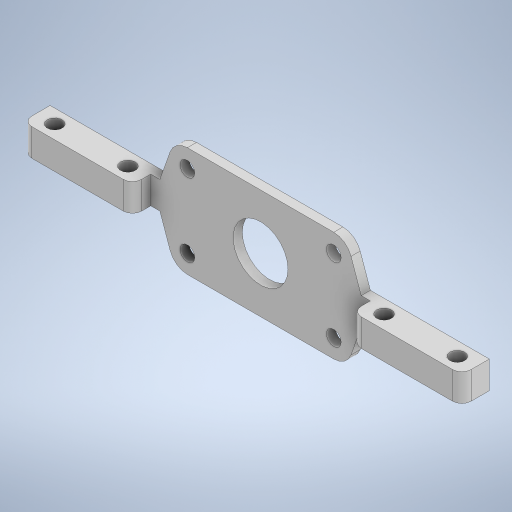
# Autodesk Inventor part: Face Plate
Saved by Autodesk Inventor 2023 (Build 270158000, 158)
## iProperties
Created: 2023-02-27
Part Number: Face Plate
Material: Generic
Document SubType Name: Modeling
Designer: Gabriel - T3 CAD
Density: 1 g/cm^3
Appearance: Default
Author: Gabriel - T3 CAD
Autodesk Inventor part; units mm, degrees
ref_plane "YZ Plane" through (0, 0, 0) normal (1, 0, 0) x (0, 1, 0)
ref_plane "XZ Plane" through (0, 0, 0) normal (0, 1, 0) x (-1, 0, 0)
ref_plane "XY Plane" through (0, 0, 0) normal (0, 0, 1) x (1, 0, 0)
sketch "Sketch1" plane through (0, 0, 0) normal (0, 1, 0) x (-1, 0, 0)
  line L0 (0, 0) -> (152.4, 0)
  line L1 (152.4, 0) -> (152.4, 6.35)
  line L2 (34.925, 9.525) -> (3.175, 9.525)
  line L3 (0, 6.35) -> (0, 0)
  circle A0 centre (6.35, 4.7625) radius 2.5797
  circle A1 centre (31.75, 4.7625) radius 2.5797
  circle A2 centre (120.65, 4.7625) radius 2.5797
  circle A3 centre (146.05, 4.7625) radius 2.5797
  line L4 (38.1, 9.525) -> (114.3, 9.525)
  line L5 (114.3, 6.35) -> (114.3, 4.7625)
  line L6 (38.1, 4.7625) -> (38.1, 6.35)
  arc A4 (38.1, 6.35) -> (34.925, 9.525) centre (34.925, 6.35) ccw
  arc A5 (3.175, 9.525) -> (0, 6.35) centre (3.175, 6.35) ccw
  line L7 (117.475, 9.525) -> (149.225, 9.525)
  arc A6 (117.475, 9.525) -> (114.3, 6.35) centre (117.475, 6.35) ccw
  arc A7 (152.4, 6.35) -> (149.225, 9.525) centre (149.225, 6.35) ccw
  line L8 (114.3, 6.35) -> (114.3, 0)
  line L9 (38.1, 6.35) -> (38.1, 0)
  line L10 (114.3, 4.7625) -> (114.3, 9.525)
  line L11 (117.475, 9.525) -> (114.3, 9.525)
  line L12 (38.1, 6.35) -> (38.1, 9.525)
  line L13 (38.1, 9.525) -> (34.925, 9.525)
  line L14 (38.1, 3.175) -> (114.3, 3.175)
  point P0 (152.4, 9.525)
  point P1 (0, 9.525)
  dimension "d0" = 152.4
  dimension "d1" = 9.525
  dimension "d2" = 4.7625
  dimension "d3" = 4.7625
  dimension "d4" = 4.7625
  dimension "d5" = 4.7625
  dimension "d6" = 25.4
  dimension "d7" = 25.4
  dimension "d8" = 5.1594
  dimension "d9" = 6.35
  dimension "d10" = 6.35
  dimension "d11" = 4.7625
  dimension "d12" = 6.35
  dimension "d13" = 6.35
  dimension "d14" = 3.175
  dimension "d15" = 3.175
  dimension "d37" = 3.175
  constraints: 30 end point, 11 point on line, 10 tangent, 8 centre point, 8 point on circle, 7 perpendicular, 5 equal radius, 3 horizontal, 3 parallel, 2 midpoint
  measures "d0" distance of point (152.4, 9.525) point (0, 9.525)
  measures "d1" distance of L0.end point (152.4, 9.525)
  measures "d2" distance from line of L0 A0.centre
  measures "d3" distance from line of L0 A1.centre
  measures "d4" distance from line of L0 A2.centre
  measures "d5" distance from line of L0 A3.centre
  measures "d6" distance of A0.centre A1.centre
  measures "d7" distance of A2.centre A3.centre
  measures "d8" diameter of A3
  measures "d9" distance from line of L3 A0.centre
  measures "d10" distance from line of L1 A3.centre
  measures "d11" distance of L6.start L4.start
  measures "d12" distance from line of A1.centre L6
  measures "d13" distance from line of A2.centre L5
  measures "d14" radius of A4
  measures "d15" radius of A6
  measures "d37" distance between parallel lines of L14 L0
extrude "Extrusion1" add sketch "Sketch1" along normal mid plane 9.525 contours L3 A5 L2 A4 L6 L9 L0 | L9 L14 L8 L0 | L8 L5 A6 L7 A7 L1 L0
extrude "Extrusion2" add sketch "Sketch1" along normal mid plane 50.8 contours L9 L14 L8 L0
sketch "Sketch3" plane through (-152.4, -4.7625, 0) normal (0, 0, -1) x (-1, 0, 0)
  line L0 (-38.1, -20.6375) -> (-38.1, 0)
  line L1 (-114.3, 30.1625) -> (-38.1, 30.1625)
  line L2 (-38.1, 30.1625) -> (-38.1, -20.6375)
  line L3 (-38.1, -20.6375) -> (-114.3, -20.6375)
  line L4 (-114.3, -20.6375) -> (-114.3, 30.1625)
  circle A0 centre (-76.2, 4.7625) radius 9.525
  line L5 (-101.6, -20.6375) -> (-101.6, 30.1625)
  line L6 (-101.6, 30.1625) -> (-50.8, 30.1625)
  line L7 (-50.8, 30.1625) -> (-50.8, -20.6375)
  line L8 (-50.8, -20.6375) -> (-101.6, -20.6375)
  line L9 (-101.6, 17.4625) -> (-50.8, 17.4625)
  line L10 (-50.8, 17.4625) -> (-50.8, -7.9375)
  line L11 (-50.8, -7.9375) -> (-101.6, -7.9375)
  line L12 (-101.6, -7.9375) -> (-101.6, 17.4625)
  circle A1 centre (-101.6, 17.4625) radius 2.5797
  circle A2 centre (-101.6, -7.9375) radius 2.5797
  circle A3 centre (-50.8, -7.9375) radius 2.5797
  circle A4 centre (-50.8, 17.4625) radius 2.5797
  circle A5 centre (-101.6, 17.4625) radius 6.35
  circle A6 centre (-101.6, -7.9375) radius 6.35
  circle A7 centre (-50.8, -7.9375) radius 6.35
  circle A8 centre (-50.8, 17.4625) radius 6.35
  line L13 (-107.95, 23.8125) -> (-44.45, 23.8125)
  line L14 (-44.45, 23.8125) -> (-44.45, -14.2875)
  line L15 (-44.45, -14.2875) -> (-107.95, -14.2875)
  line L16 (-107.95, -14.2875) -> (-107.95, 23.8125)
  line L17 (-114.3, 9.525) -> (-117.475, 9.525)
  line L18 (-114.3, 0) -> (-114.3, 9.525)
  line L19 (-38.1, 0) -> (-38.1, 9.525)
  line L20 (-114.3, 9.525) -> (-107.95, 9.525)
  line L21 (-111.125, 9.525) -> (-101.3931, 37.1795)
  line L22 (-114.3, 0) -> (-114.3, 9.525)
  line L23 (-114.3, 0) -> (-107.95, 0)
  line L24 (-111.125, 0) -> (-100.7566, -29.4634)
  line L25 (-38.1, 0) -> (-44.45, 0)
  line L26 (-38.1, 9.525) -> (-38.1, 30.1625)
  line L27 (-38.1, 9.525) -> (-44.45, 9.525)
  line L28 (-41.275, 9.525) -> (-52.247, 40.7036)
  line L29 (-41.275, 0) -> (-51.6214, -29.4007)
  line L30 (0, 0) -> (-38.1, 0) projected
  line L31 (-114.3, 9.525) -> (-114.3, 30.1625) projected
  point P0 (-152.4, 4.7625)
  point P1 (-41.275, 0)
  point P2 (-107.5899, 19.5704)
  point P3 (-101.6, 23.8125)
  point P4 (-50.8, 23.8125)
  point P5 (-44.8101, 19.5704)
  point P6 (-38.1, 0)
  point P7 (-44.8101, -10.0454)
  point P8 (-50.8, -14.2875)
  point P9 (-101.6, -14.2875)
  point P10 (-107.5899, -10.0454)
  dimension "d38" = 25.4
  dimension "d39" = 38.1
  dimension "d40" = 50.8
  dimension "d41" = 25.4
  dimension "d42" = 12.7
  dimension "d43" = 19.05
  dimension "d44" = 5.1594
  dimension "d45" = 12.7
  dimension "d46" = 12.7
  dimension "d47" = 12.7
  dimension "d48" = 12.7
  dimension "d49" = 160.613
  dimension "d50" = 160.613
  dimension "d51" = 6.35
  dimension "d52" = 76.2
  dimension "d53" = 30.1625
  dimension "d54" = 13.5214
  dimension "d55" = 14.147
  dimension "d56" = 62.6566
  dimension "d57" = 63.2931
  dimension "d58" = 79.375
  constraints: 60 end point, 11 parallel, 10 coincident, 9 centre point, 8 perpendicular, 8 point on line, 8 tangent, 4 midpoint, 3 equal radius, 3 horizontal, 1 vertical, 9 other
  measures "d38" distance from line of L1 A0.centre
  measures "d39" distance from line of L4 A0.centre
  measures "d40" distance of L6.start L6.end
  measures "d41" distance between parallel lines of L11 L9
  measures "d42" distance between parallel lines of L6 L9
  measures "d43" diameter of A0
  measures "d44" diameter of A1
  measures "d45" diameter of A5
  measures "d46" diameter of A6
  measures "d47" diameter of A7
  measures "d48" diameter of A8
  measures "d49" angle of L26 L29
  measures "d50" angle of L0 L28
  measures "d51" distance between parallel lines of L2 L14
  measures "d52" distance between parallel lines of L2 L22
  measures "d53" distance between parallel lines of L27 L3
  measures "d54" distance from line of L29.end L2
  measures "d55" distance from line of L28.end L2
  measures "d56" distance from line of L24.end L2
  measures "d57" distance from line of L21.end L2
  measures "d58" distance from line of L17.end L2
extrude "Extrusion4" cut sketch "Sketch3" against normal blind 50.8 contours L3 L29 L15 L14 L25 L0 | L3 L7 L15 L29 | L27 L28 L14 L13 L1 L2 | L3 L5 L15 L7 | L29 L14 L15 | L15 A7 L29 | L3 L24 L15 L5 | L28 L13 L7 L1 | L28 L13 L14 | L3 L4 L23 L24 L16 L15 | L15 L24 A6 | A3 L11 L7 | L7 A3 | L7 L13 L5 L1 | L28 A8 L13 | L15 L16 L24 | A2 L5 | L5 L11 A2 | L11 A3 L7 | L5 L13 L21 L1 | L5 A2 L11 | L21 L13 L16 L20 L4 L1 | A5 L21 L13 | A4 L7 | L7 L9 A4 | A4 L9 L7 | L21 L16 L13 | A1 L9 L5 | L5 A1 | L5 L9 A1 | A0
equation "\"d2\" = 0.5 * d1"
equation "\"d3\" = d2"
equation "\"d4\" = d2"
equation "\"d5\" = d2"
equation "\"d10\" = d9"
equation "\"d11\" = 0.5 * d1"
equation "\"d37\" = 0.333333 * d1"
body "Solid1"
